small screen insert_v1 (Autodesk Fusion 360 design; units mm, degrees)
Autodesk Fusion 360 part; units mm, degrees
sketch "Esquisse1" plane through (0, 0, 0) normal (0, 0, 1) x (1, 0, 0)
  line L0 (13.5, 8) -> (-13.5, 8)
  line L1 (-13.5, 8) -> (-13.5, -8)
  line L2 (-13.5, -8) -> (13.5, -8)
  line L3 (13.5, -8) -> (13.5, 8)
  line L4 (13.5, 8) -> (-13.5, -8) construction
  line L5 (-13.5, 8) -> (13.5, -8) construction
  line L6 (13.75, 13.95) -> (-13.75, 13.95)
  line L7 (-13.75, 13.95) -> (-13.75, -13.95)
  line L8 (-13.75, -13.95) -> (13.75, -13.95)
  line L9 (13.75, -13.95) -> (13.75, 13.95)
  line L10 (13.75, 13.95) -> (-13.75, -13.95) construction
  line L11 (-13.75, 13.95) -> (13.75, -13.95) construction
  line L12 (-16.75, -16.95) -> (16.75, -16.95)
  line L13 (16.75, -16.95) -> (16.75, 16.95)
  line L14 (16.75, 16.95) -> (-16.75, 16.95)
  line L15 (-16.75, 16.95) -> (-16.75, -16.95)
  dimension "d1" = 27
  dimension "d2" = 16
  dimension "d3" = 27.5
  dimension "d4" = 27.9
  dimension "d5" = 3
  constraint horizontal L0
  constraint perpendicular L0 L1
  constraint parallel L0 L2
  constraint parallel L1 L3
  constraint coincident L4 origin
  constraint coincident L5 origin
  constraint horizontal L6
  constraint perpendicular L6 L7
  constraint parallel L6 L8
  constraint parallel L7 L9
  constraint coincident L10 origin
  constraint coincident L11 origin
  measures "d1" distance of L1.end L2.end
  measures "d2" distance of L0.end L1.end
  measures "d3" distance of L7.end L8.end
  measures "d4" distance of L6.end L7.end
extrude "Extrusion1" add sketch "Esquisse1" along normal blind 3.6 contours L6 L7 L8 L9
extrude "Extrusion2" add sketch "Esquisse1" along normal blind 5.6 contours L12 L13 L14 L15
extrude "Extrusion3" cut sketch "Esquisse1" along normal blind 2.6 contours L12 L13 L14 L15
equation "d6 = 2.6 mm + 1 mm"
equation "d8 = 2.6 mm + 3 mm"
